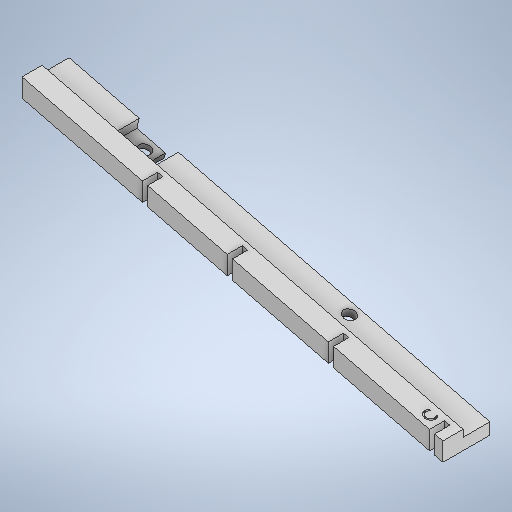
# Autodesk Inventor part: Commodore Left mount
Saved by Autodesk Inventor 2025 (Build 290162000, 162)
## iProperties
Created: 2024-07-17
Part Number: Commodore Left mount
Material: Generic
Document SubType Name: Modeling
Designer: adam
Density: 1 g/cm^3
Appearance: Default
Author: adam
Autodesk Inventor part; units mm, degrees
ref_plane "YZ Plane" through (0, 0, 0) normal (1, 0, 0) x (0, 1, 0)
ref_plane "XZ Plane" through (0, 0, 0) normal (0, 1, 0) x (-1, 0, 0)
ref_plane "XY Plane" through (0, 0, 0) normal (0, 0, 1) x (1, 0, 0)
sketch "Sketch1" plane through (0, 0, 0) normal (0, 0, 1) x (1, 0, 0)
  line L0 (0, 0) -> (-125.1681, 31.2079)
  line L1 (0, 0) -> (-48.3113, 0) construction
  line L2 (0, 0) -> (0, 5.5)
  line L3 (-125.1681, 31.2079) -> (-125.1681, 36.7079)
  line L4 (-125.1681, 36.7079) -> (0, 5.5)
  dimension "d0" = 14
  dimension "d1" = 129
  dimension "d2" = 5.5
  dimension "d3" = 5.5
  constraints: 10 end point, 1 horizontal, 1 perpendicular, 1 vertical
  measures "d0" angle of L1 L0
  measures "d1" distance of L0.start L0.end
  measures "d2" distance of L0.start L2.end
  measures "d3" distance of L0.end L3.end
extrude "Side rail" add sketch "Sketch1" against normal blind 6
sketch "Sketch2" plane through (0, 0, 0) normal (0, 0, 1) x (1, 0, 0)
  line L0 (-125.1681, 36.7079) -> (0, 5.5) projected
  line L1 (-2.4257, 6.1048) -> (-2.4257, 0.6048)
  line L2 (0, 0) -> (-125.1681, 31.2079) projected
  line L3 (0, 5.5) -> (-125.1681, 36.7079) construction
  line L4 (-125.1681, 36.7079) -> (-125.1681, 31.2079) construction
  line L5 (-125.1681, 31.2079) -> (0, 0) construction
  line L6 (0, 0) -> (0, 5.5) construction
  line L7 (-2.4257, 6.1048) -> (-3.9757, 6.4913)
  line L8 (-3.9757, 6.4913) -> (-3.9757, 0.9913)
  line L9 (-3.9757, 0.9913) -> (-2.4257, 0.6048)
  line L10 (-32.5049, 8.1044) -> (-34.0549, 8.4908)
  line L11 (-34.0549, 13.9908) -> (-32.5049, 13.6044)
  line L12 (-60.2529, 20.5227) -> (-58.7029, 20.1363)
  line L13 (-2.4257, 6.1048) -> (-3.9757, 6.1048) construction
  line L14 (-84.9009, 21.1682) -> (-86.4509, 21.5546)
  line L15 (-86.4509, 27.0546) -> (-84.9009, 26.6682)
  line L16 (0, 5.5) -> (-125.1681, 36.7079) projected
  line L17 (-125.1681, 31.2079) -> (0, 0) projected
  line L18 (-32.5049, 13.6044) -> (-32.5049, 8.1044)
  line L19 (-34.0549, 13.9908) -> (-34.0549, 8.4908)
  line L20 (-62.5841, 21.104) -> (-62.5841, 15.604)
  line L21 (-64.1341, 21.4904) -> (-64.1341, 15.9904)
  line L22 (-87.8118, 27.3939) -> (-87.8118, 21.8939)
  line L23 (-89.3618, 27.7804) -> (-89.3618, 22.2804)
  line L24 (-87.8118, 27.3939) -> (-89.3618, 27.3939) construction
  line L25 (-62.5841, 21.104) -> (-64.1341, 21.104) construction
  line L26 (-32.5049, 13.6044) -> (-34.0549, 13.6044) construction
  point P0 (-3.9757, 0.9913)
  point P1 (-34.0549, 13.9908)
  point P2 (-34.0549, 8.4908)
  point P3 (-32.5049, 8.1044)
  point P4 (-32.5049, 13.6044)
  point P5 (-64.1341, 21.4904)
  point P6 (-64.1341, 15.9904)
  point P7 (-62.5841, 15.604)
  point P8 (-89.3618, 22.2804)
  point P9 (-87.8118, 21.8939)
  point P10 (-87.8118, 27.3939)
  dimension "d6" = 1.55
  dimension "d7" = 2.5
  dimension "d43" = 88
  dimension "d44" = 62
  dimension "d45" = 31
  constraints: 38 end point, 14 point on line, 6 parallel, 5 collinear, 5 vertical, 3 perpendicular, 14 other
  measures "d6" distance of L1.start L13.end
  measures "d7" distance of L2.start L1.end
  measures "d43" distance of L1.end L22.end
  measures "d44" distance of L1.end L20.end
  measures "d45" distance of L1.end L18.end
extrude "Side rail cuts" cut sketch "Sketch2" against normal blind 4.5 contours L0 L22 L2 L23 | L0 L20 L2 L21 | L19 L0 L18 L2 | L8 L0 L1 L2
sketch "Sketch3" plane through (0, 0, -6) normal (0, 0, -1) x (-1, 0, 0)
  line L0 (0, 0) -> (125.1681, 31.2079) projected
  line L1 (0, 0) -> (0, 5.5) projected
  line L2 (0, 3.4388) -> (125.1681, 34.6467)
  line L3 (125.1681, 36.7079) -> (125.1681, 31.2079) projected
  line L4 (0, 3.4388) -> (0, 0)
  line L5 (125.1681, 34.6467) -> (125.1681, 31.2079)
  line L6 (125.1681, 36.7079) -> (0, 5.5) projected
  dimension "d12" = 2
  constraints: 6 end point, 2 collinear, 2 point on line
  measures "d12" distance between parallel lines of L2 L6
extrude "Keyboard support" add sketch "Sketch3" along normal blind 8 contours L1 L2 L3 L0
sketch "Sketch4" plane through (0, 3.4388, -6) normal (0.2419219, 0.9702957, 0) x (0.9702957, -0.2419219, 0)
  line L0 (-129, 0) -> (-129, 8) construction
  line L1 (-129, 5) -> (0, 5) construction
  line L2 (0, 0) -> (0, 8) construction
  line L3 (0, 0) -> (-129, 0) construction
  circle A0 centre (-40, 5) radius 1.75
  line L4 (0.8319, 8) -> (-128.1681, 8) projected
  line L5 (-95.5, 8) -> (-95.5, 0)
  line L6 (-107.5, 0) -> (-107.5, 8)
  line L7 (-107.5, 8) -> (-95.5, 8)
  line L8 (-107.5, 0) -> (-95.5, 0)
  point P0 (0.8319, -6)
  dimension "d16" = 5
  dimension "d17" = 40
  dimension "d18" = 95.5
  dimension "d19" = 12
  dimension "d20" = 3.5
  constraints: 10 end point, 7 point on line, 2 collinear, 2 perpendicular, 1 centre point, 1 horizontal
  measures "d16" distance between parallel lines of L1 L3
  measures "d17" distance from line of L2 A0.centre
  measures "d18" distance between parallel lines of L2 L5
  measures "d19" distance between parallel lines of L5 L6
  measures "d20" diameter of A0
extrude "Mount hole and brace clearance" cut sketch "Sketch4" against normal up to surface (3.3366 mm away)
sketch "Sketch5" plane through (0, 0, -6) normal (0, 0, -1) x (-1, 0, 0)
  line L0 (125.1681, 34.6467) -> (104.3068, 29.4454) construction
  line L1 (104.3068, 29.4454) -> (92.6269, 26.5333) construction
  line L2 (104.3068, 29.4454) -> (105.114, 26.2079) projected
  line L3 (105.0326, 26.5345) -> (96.494, 24.4056)
  line L4 (96.494, 24.4056) -> (96.8568, 22.9501)
  line L5 (96.8568, 22.9501) -> (111.4113, 26.579)
  line L6 (111.4113, 26.579) -> (111.0484, 28.0344)
  line L7 (111.0484, 28.0344) -> (105.0326, 26.5345)
  line L8 (93.4704, 23.3048) -> (92.6632, 26.5423) projected
  point P0 (0, 0)
  dimension "d23" = 3
  dimension "d24" = 1.5
  dimension "d25" = 3.2
  dimension "d26" = 15
  constraints: 12 end point, 4 perpendicular, 1 collinear, 1 point on line
  measures "d23" distance between parallel lines of L3 L1
  measures "d24" distance between parallel lines of L5 L3
  measures "d25" distance between parallel lines of L4 L8
  measures "d26" distance between parallel lines of L6 L4
extrude "Brace support" add sketch "Sketch5" along normal blind 8 and the other way blind 3.3
sketch "Sketch6" plane through (-96.494, 24.4056, -6) normal (0.2419219, 0.9702957, 0) x (0.9702957, -0.2419219, 0)
  circle A0 centre (-3.3, 5) radius 1.75
  circle A1 centre (58.7, 5) radius 1.75 construction
  line L0 (-30.7987, 0) -> (98.2013, 0) construction
  line L1 (98.7, 0) -> (98.7, 8) construction
  point P0 (99.5319, -6)
  dimension "d31" = 5
  dimension "d32" = 102
  constraints: 1 centre point, 1 equal radius
  measures "d31" distance from line of A0.centre L0
  measures "d32" distance from line of L1 A0.centre
extrude "Extrusion6" cut sketch "Sketch6" against normal up to surface (1.5 mm away)
sketch "Sketch8" plane through (0, 0, -14) normal (-0.2419219, -0.9702957, 0) x (0.9702957, -0.2419219, 0)
  circle A0 centre (-40.8319, 3) radius 1.75 projected
  arc A1 (-37.0819, 3) -> (-44.5819, 3) centre (-40.8319, 3) ccw
  line L0 (0, 0) -> (-96.3319, 0) projected
  line L1 (-37.0819, 3) -> (-37.0819, 0)
  line L2 (-44.5819, 3) -> (-44.5819, 0)
  point P0 (0, 14)
  dimension "d40" = 7.5
  constraints: 4 end point, 2 perpendicular, 2 point on circle, 2 point on line, 2 tangent, 1 centre point, 1 coincident
  measures "d40" diameter of A1
extrude "Extrusion8" cut sketch "Sketch8" against normal blind 1
sketch "Sketch9" plane through (0, 5.5, 0) normal (0.2419219, 0.9702957, 0) x (0.9702957, -0.2419219, 0)
  line L0 (-8.6927, 1.2346) -> (-8.6927, 4.3985) construction
  line L1 (-8.6927, 4.3985) -> (-5.5693, 4.3985) construction
  line L2 (-5.5693, 4.3985) -> (-5.5693, 1.2346) construction
  line L3 (-5.5693, 1.2346) -> (-8.6927, 1.2346) construction
  line L4 (-4.0975, 0) -> (-33.5, 0) projected
  line L5 (-6.3134, 4.1985) -> (-5.8325, 4.1985)
  spline S0 degree 2 poles (-5.8325, 4.1985) (-5.5693, 3.7176) (-5.5693, 3.0899) knots 0 0 0 1 1 1
  spline S1 degree 2 poles (-5.5693, 3.0899) (-5.5693, 2.5786) (-5.9793, 1.8673) (-6.7007, 1.4522) (-7.1183, 1.4522) knots 0 0 0 1 2 3 3 3
  spline S2 degree 2 poles (-7.1183, 1.4522) (-7.784, 1.4522) (-8.6927, 2.4014) (-8.6927, 3.0975) knots 0 0 0 1 2 2 2
  spline S3 degree 2 poles (-8.6927, 3.0975) (-8.6927, 3.5784) (-8.4396, 4.1656) knots 0 0 0 1 1 1
  line L6 (-8.4396, 4.1656) -> (-7.9713, 4.1656)
  spline S4 degree 2 poles (-7.9713, 4.1656) (-8.2776, 3.6315) (-8.2776, 3.1203) knots 0 0 0 1 1 1
  spline S5 degree 2 poles (-8.2776, 3.1203) (-8.2776, 2.5963) (-7.6169, 1.9053) (-7.1183, 1.9053) knots 0 0 0 1 2 2 2
  spline S6 degree 2 poles (-7.1183, 1.9053) (-6.6172, 1.9053) (-5.9717, 2.5862) (-5.9717, 3.1152) knots 0 0 0 1 2 2 2
  spline S7 degree 2 poles (-5.9717, 3.1152) (-5.9717, 3.6695) (-6.3134, 4.1985) knots 0 0 0 1 1 1
  point P0 (1.3306, 0)
  constraints: 1 parallel, 2 other
extrude "Extrusion9" cut sketch "Sketch9" against normal blind 0.5
body "Solid1"
